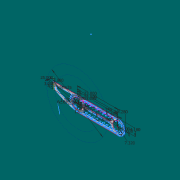
# Autodesk Inventor part: TG2
Saved by Autodesk Inventor 2016 (Build 200138000, 138)
## iProperties
Created: 2017-06-03
Part Number: TG2
Material: Aluminum 6061
Document SubType Name: Sheet Metal
Designer: katzchristy
Density: 2.7 g/cm^3
Appearance: Aluminum - Flat
Sheet Metal Rule: Default
Author: katzchristy
Autodesk Inventor part; units mm, degrees
ref_plane "YZ Plane" through (0, 0, 0) normal (1, 0, 0) x (0, 1, 0)
ref_plane "XZ Plane" through (0, 0, 0) normal (0, 1, 0) x (-1, 0, 0)
ref_plane "XY Plane" through (0, 0, 0) normal (0, 0, 1) x (1, 0, 0)
sketch "Fender Base" plane through (0, 0, 0) normal (0, 0, 1) x (1, 0, 0)
  line L0 (-7.62, 106.172) -> (7.62, 106.172) construction
  line L1 (111.252, 7.62) -> (111.252, -7.62)
  line L2 (576.58, 106.172) -> (591.82, 106.172) construction
  line L3 (692.912, 7.62) -> (692.912, -7.62) construction
  line L4 (-7.62, 106.172) -> (591.82, 106.172)
  arc A0 (528.4894, 74.422) -> (584.2, 92.964) centre (584.2, 0) ccw construction
  circle A1 centre (0, 0) radius 92.964 construction
  arc A2 (584.2, -106.4451) -> (591.82, 106.172) centre (584.2, 0) ccw
  line L5 (584.2, 0) -> (584.2, -74.422) construction
  line L6 (0, 0) -> (0, -106.4451) construction
  line L7 (0, -106.4451) -> (584.2, -106.4451)
  line L8 (0, 92.964) -> (584.2, 92.964) construction
  line L9 (0, -92.964) -> (584.2, -92.964) construction
  line L10 (75.7223, 74.422) -> (508.4777, 74.422)
  line L11 (0, 0) -> (584.2, 0) construction
  line L12 (75.7223, -74.422) -> (508.4777, -74.422)
  arc A3 (0, -74.422) -> (0, 74.422) centre (0, 0) ccw
  arc A4 (509.778, 0) -> (584.2, -74.422) centre (584.2, 0) ccw
  arc A5 (0, 74.422) -> (0, -74.422) centre (0, 0) ccw
  line L13 (584.2, -74.422) -> (584.2, -106.4451) construction
  arc A6 (584.2, 74.422) -> (509.778, 0) centre (584.2, 0) ccw
  arc A7 (584.2, -74.422) -> (584.2, 74.422) centre (584.2, 0) ccw
  arc A8 (479.2215, -15.875) -> (508.4777, -74.422) centre (584.2, 0) ccw
  arc A9 (508.4777, 74.422) -> (479.2215, 15.875) centre (584.2, 0) ccw
  arc A10 (584.2, 92.964) -> (528.4894, 74.422) centre (584.2, 0) ccw construction
  line L14 (104.9785, 15.875) -> (479.2215, 15.875)
  line L15 (104.9785, -15.875) -> (479.2215, -15.875)
  arc A11 (75.7223, -74.422) -> (104.9785, -15.875) centre (0, 0) ccw
  arc A12 (104.9785, 15.875) -> (75.7223, 74.422) centre (0, 0) ccw
  line L16 (111.252, 7.62) -> (111.252, -7.62) construction
  circle A13 centre (0, 0) radius 78.74 construction
  circle A14 centre (-433.085, 76.2) radius 38.1 construction
  circle A15 centre (0, 0) radius 439.7375 construction
  circle A16 centre (-306.5807, 82.55) radius 3.175 construction
  arc A17 (-317.4589, 5.1115) -> (-308.6545, 74.422) centre (0, 0) ccw construction
  line L17 (-429.979, 114.1732) -> (6.4191, 78.4779) construction
  line L18 (-443.1268, 39.4471) -> (-20.753, -75.9559) construction
  line L19 (-7.62, 106.172) -> (-347.8163, 106.172)
  line L20 (-347.8163, 155.9143) -> (-347.8163, -18.2544) construction
  arc A18 (-321.9776, 6.3462) -> (-34.5848, -100.67) centre (194.8237, 954.8143) ccw
  line L21 (-347.8163, 106.172) -> (-321.9776, 6.3462)
  line L22 (-283.1615, -143.6169) -> (-252.5039, -262.0603)
  arc A19 (-294.7226, 27.7545) -> (-91.9832, -53.5691) centre (194.8237, 954.8143) ccw
  line L23 (-294.7226, 27.7545) -> (-306.8019, 74.422)
  line L24 (-306.8019, 74.422) -> (-76.1047, 74.422)
  arc A20 (-76.1047, 74.422) -> (-91.9832, -53.5691) centre (0, 0) ccw
  arc A21 (-34.5848, -100.67) -> (0, -106.4451) centre (0, 0) ccw
  point P0 (0, 106.172)
  point P1 (111.252, 0)
  point P2 (584.2, 106.172)
  point P3 (692.912, 0)
  dimension "d100" = 879.475
  dimension "d0" = 15.24
  dimension "d1" = 106.172
  dimension "d2" = 15.24
  dimension "d3" = 111.252
  dimension "d4" = 15.24
  dimension "d5" = 106.172
  dimension "d6" = 584.2
  dimension "d7" = 15.24
  dimension "d8" = 108.712
  dimension "d9" = 584.2
  dimension "d10" = 185.928
  dimension "d11" = 185.928
  dimension "d13" = 584.2
  dimension "d14" = 31.75
  dimension "d66" = 31.75
  dimension "d96" = 157.48
  dimension "d97" = 76.2
  dimension "d99" = 76.2
  dimension "d101" = 6.35
  dimension "d102" = 82.55
  dimension "d103" = 635
  dimension "d106" = 31.75
  constraints: 50 end point, 43 point on circle, 21 centre point, 9 coincident, 8 point on line, 7 horizontal, 6 vertical, 5 tangent, 4 midpoint, 3 horizontal alignment, 2 equal length, 2 symmetric about line, 2 vertical alignment, 4 other
  measures "d0" distance of L0.start L0.end
  measures "d1" distance from line of point (0, 0) L0
  measures "d2" distance of L1.start L1.end
  measures "d3" distance from line of point (0, 0) L1
  measures "d4" distance of L2.start L2.end
  measures "d5" distance from line of point (0, 0) L2
  measures "d6" horizontal distance of point (0, 0) point (584.2, 106.172)
  measures "d7" distance of L3.start L3.end
  measures "d8" distance from line of L3 point (584.2, 0)
  measures "d9" distance of point (584.2, 0) point (0, 0)
  measures "d10" diameter of A0
  measures "d11" diameter of A1
  measures "d13" distance of A3.end A6.start
  measures "d14" distance between parallel lines of L10 L2
  measures "d66" distance between parallel lines of L15 L14
  measures "d96" diameter of A13
  measures "d97" diameter of A14
  measures "d99" vertical distance of point (0, 0) A14.centre
  measures "d101" diameter of A16
  measures "d102" vertical distance of point (0, 0) A16.centre
  measures "d103" diameter of A17
  measures "d106" radial gap between concentric circles of A18 A19
extrude "Plate1" add sketch "Fender Base" along normal blind 1.6281 contours L4 A2 L7 A21 A18 L21 L19 | L10 A9 L14 A12 | A5 A3 | A6 A7 A4 | L23 L24 A20 A19
sketch "Oval Pattern" plane through (0, 0, 1.6281) normal (0, 0, 1) x (1, 0, 0)
  circle A0 centre (-25.6073, 82.042) radius 6.35
  arc A1 (-14.4463, 83.0479) -> (-28.9236, 92.7462) centre (-25.6073, 82.042) ccw
  arc A2 (12.2648, 98.9975) -> (-28.9236, 92.7462) centre (-1.2605, 49.2962) ccw
  arc A3 (12.2648, 98.9975) -> (-14.4463, 83.0479) centre (17.7837, 59.4132) ccw
  circle A4 centre (-61.4767, 60.0603) radius 6.35
  arc A5 (-52.1303, 66.2426) -> (-69.4759, 67.9082) centre (-61.4767, 60.0603) ccw
  arc A6 (-36.1888, 92.9586) -> (-69.4759, 67.9082) centre (-24.5055, 42.7924) ccw
  arc A7 (-36.1888, 92.9586) -> (-52.1303, 66.2426) centre (-12.5443, 60.7357) ccw
  circle A8 centre (-82.6165, 23.6883) radius 6.35
  arc A9 (-77.3239, 33.5658) -> (-93.3821, 26.7996) centre (-82.6165, 23.6883) ccw
  arc A10 (-75.9716, 64.6471) -> (-93.3821, 26.7996) centre (-41.879, 26.0356) ccw
  arc A11 (-75.9716, 64.6471) -> (-77.3239, 33.5658) centre (-39.8667, 47.5062) ccw
  circle A12 centre (-83.9616, -18.3594) radius 6.35
  arc A13 (-83.991, -7.1533) -> (-94.9141, -20.7301) centre (-83.9616, -18.3594) ccw
  arc A14 (-97.5518, 20.8463) -> (-94.9141, -20.7301) centre (-49.2185, 3.0408) ccw
  arc A15 (-97.5518, 20.8463) -> (-83.991, -7.1533) centre (-57.6371, 22.8943) ccw
  circle A16 centre (-65.1898, -56.0082) radius 6.35
  arc A17 (-70.534, -46.1585) -> (-73.705, -63.293) centre (-65.1898, -56.0082) ccw
  arc A18 (-95.7589, -27.9492) -> (-73.705, -63.293) centre (-44.7653, -20.6826) ccw
  arc A19 (-95.7589, -27.9492) -> (-70.534, -46.1585) centre (-61.5979, -7.2031) ccw
  circle A20 centre (-30.7986, -80.2376) radius 6.35
  arc A21 (-40.1773, -74.1042) -> (-34.8364, -90.691) centre (-30.7986, -80.2376) ccw
  arc A22 (-71.0224, -70.0481) -> (-34.8364, -90.691) centre (-29.5865, -39.4505) ccw
  arc A23 (-71.0224, -70.0481) -> (-40.1773, -74.1042) centre (-50.8, -35.5745) ccw
  circle A24 centre (10.9718, -85.2423) radius 6.35
  arc A25 (-0.1943, -84.2948) -> (12.3789, -96.3597) centre (10.9718, -85.2423) ccw
  arc A26 (-29.2692, -95.3637) -> (12.3789, -96.3597) centre (-7.3189, -48.7662) ccw
  arc A27 (-29.2692, -95.3637) -> (-0.1943, -84.2948) centre (-27.8305, -55.4225) ccw
  line L0 (-347.8163, 106.172) -> (591.82, 106.172) projected
  circle A28 centre (19.9908, 83.9489) radius 6.35
  arc A29 (31.1517, 84.9548) -> (16.6745, 94.6531) centre (19.9908, 83.9489) ccw
  arc A30 (57.8628, 100.9043) -> (16.6745, 94.6531) centre (44.3376, 51.2031) ccw
  arc A31 (57.8628, 100.9043) -> (31.1517, 84.9548) centre (63.3817, 61.32) ccw
  circle A32 centre (65.7108, 83.9489) radius 6.35
  arc A33 (76.8717, 84.9548) -> (62.3945, 94.6531) centre (65.7108, 83.9489) ccw
  arc A34 (103.5828, 100.9043) -> (76.8717, 84.9548) centre (109.1017, 61.32) ccw
  arc A35 (103.5828, 100.9043) -> (62.3945, 94.6531) centre (90.0576, 51.2031) ccw
  circle A36 centre (111.4308, 83.9489) radius 6.35
  arc A37 (122.5917, 84.9548) -> (108.1145, 94.6531) centre (111.4308, 83.9489) ccw
  arc A38 (149.3028, 100.9043) -> (122.5917, 84.9548) centre (154.8217, 61.32) ccw
  arc A39 (149.3028, 100.9043) -> (108.1145, 94.6531) centre (135.7776, 51.2031) ccw
  circle A40 centre (157.1508, 83.9489) radius 6.35
  arc A41 (168.3117, 84.9548) -> (153.8345, 94.6531) centre (157.1508, 83.9489) ccw
  arc A42 (195.0228, 100.9043) -> (168.3117, 84.9548) centre (200.5417, 61.32) ccw
  arc A43 (195.0228, 100.9043) -> (153.8345, 94.6531) centre (181.4976, 51.2031) ccw
  circle A44 centre (202.8708, 83.9489) radius 6.35
  arc A45 (214.0317, 84.9548) -> (199.5545, 94.6531) centre (202.8708, 83.9489) ccw
  arc A46 (240.7428, 100.9043) -> (214.0317, 84.9548) centre (246.2617, 61.32) ccw
  arc A47 (240.7428, 100.9043) -> (199.5545, 94.6531) centre (227.2176, 51.2031) ccw
  circle A48 centre (248.5908, 83.9489) radius 6.35
  arc A49 (259.7517, 84.9548) -> (245.2745, 94.6531) centre (248.5908, 83.9489) ccw
  arc A50 (286.4628, 100.9043) -> (259.7517, 84.9548) centre (291.9817, 61.32) ccw
  arc A51 (286.4628, 100.9043) -> (245.2745, 94.6531) centre (272.9376, 51.2031) ccw
  circle A52 centre (294.3108, 83.9489) radius 6.35
  arc A53 (305.4717, 84.9548) -> (290.9945, 94.6531) centre (294.3108, 83.9489) ccw
  arc A54 (332.1828, 100.9043) -> (305.4717, 84.9548) centre (337.7017, 61.32) ccw
  arc A55 (332.1828, 100.9043) -> (290.9945, 94.6531) centre (318.6576, 51.2031) ccw
  circle A56 centre (340.0308, 83.9489) radius 6.35
  arc A57 (351.1917, 84.9548) -> (336.7145, 94.6531) centre (340.0308, 83.9489) ccw
  arc A58 (377.9028, 100.9043) -> (351.1917, 84.9548) centre (383.4217, 61.32) ccw
  arc A59 (377.9028, 100.9043) -> (336.7145, 94.6531) centre (364.3776, 51.2031) ccw
  circle A60 centre (385.7508, 83.9489) radius 6.35
  arc A61 (396.9117, 84.9548) -> (382.4345, 94.6531) centre (385.7508, 83.9489) ccw
  arc A62 (423.6228, 100.9043) -> (396.9117, 84.9548) centre (429.1417, 61.32) ccw
  arc A63 (423.6228, 100.9043) -> (382.4345, 94.6531) centre (410.0976, 51.2031) ccw
  circle A64 centre (431.4708, 83.9489) radius 6.35
  arc A65 (442.6317, 84.9548) -> (428.1545, 94.6531) centre (431.4708, 83.9489) ccw
  arc A66 (469.3428, 100.9043) -> (442.6317, 84.9548) centre (474.8617, 61.32) ccw
  arc A67 (469.3428, 100.9043) -> (428.1545, 94.6531) centre (455.8176, 51.2031) ccw
  circle A68 centre (477.1908, 83.9489) radius 6.35
  arc A69 (488.3517, 84.9548) -> (473.8745, 94.6531) centre (477.1908, 83.9489) ccw
  arc A70 (515.0628, 100.9043) -> (488.3517, 84.9548) centre (520.5817, 61.32) ccw
  arc A71 (515.0628, 100.9043) -> (473.8745, 94.6531) centre (501.5376, 51.2031) ccw
  circle A72 centre (522.9108, 83.9489) radius 6.35
  arc A73 (534.0717, 84.9548) -> (519.5945, 94.6531) centre (522.9108, 83.9489) ccw
  arc A74 (560.7828, 100.9043) -> (534.0717, 84.9548) centre (566.3017, 61.32) ccw
  arc A75 (560.7828, 100.9043) -> (519.5945, 94.6531) centre (547.2576, 51.2031) ccw
  circle A76 centre (568.6308, 83.9489) radius 6.35
  arc A77 (579.7917, 84.9548) -> (565.3145, 94.6531) centre (568.6308, 83.9489) ccw
  arc A78 (606.5028, 100.9043) -> (579.7917, 84.9548) centre (612.0217, 61.32) ccw
  arc A79 (606.5028, 100.9043) -> (565.3145, 94.6531) centre (592.9776, 51.2031) ccw
  line L1 (75.7223, 74.422) -> (508.4777, 74.422) projected
  circle A80 centre (612.6911, 80.4865) radius 6.35
  arc A81 (622.8597, 75.7771) -> (615.1712, 91.4147) centre (612.6911, 80.4865) ccw
  arc A82 (653.967, 76.2343) -> (615.1712, 91.4147) centre (617.4031, 39.9544) ccw
  arc A83 (653.967, 76.2343) -> (622.8597, 75.7771) centre (638.9544, 39.1938) ccw
  circle A84 centre (649.1172, 55.4578) radius 6.35
  arc A85 (655.5688, 46.2951) -> (656.7292, 63.6819) centre (649.1172, 55.4578) ccw
  arc A86 (682.7371, 31.1374) -> (656.7292, 63.6819) centre (632.9319, 17.9999) ccw
  arc A87 (682.7371, 31.1374) -> (655.5688, 46.2951) centre (651.2156, 6.5657) ccw
  circle A88 centre (668.1489, 15.5692) radius 6.35
  arc A89 (669.1548, 4.4083) -> (678.8531, 18.8855) centre (668.1489, 15.5692) ccw
  arc A90 (685.1043, -22.3028) -> (678.8531, 18.8855) centre (635.4031, -8.7776) ccw
  arc A91 (685.1043, -22.3028) -> (669.1548, 4.4083) centre (645.52, -27.8217) ccw
  circle A92 centre (664.6865, -28.4911) radius 6.35
  arc A93 (659.9771, -38.6597) -> (675.6147, -30.9712) centre (664.6865, -28.4911) ccw
  arc A94 (660.4343, -69.767) -> (675.6147, -30.9712) centre (624.1544, -33.2031) ccw
  arc A95 (660.4343, -69.767) -> (659.9771, -38.6597) centre (623.3938, -54.7544) ccw
  circle A96 centre (639.6578, -64.9172) radius 6.35
  arc A97 (630.4951, -71.3688) -> (647.8819, -72.5292) centre (639.6578, -64.9172) ccw
  arc A98 (615.3374, -98.5371) -> (647.8819, -72.5292) centre (602.1999, -48.7319) ccw
  arc A99 (615.3374, -98.5371) -> (630.4951, -71.3688) centre (590.7657, -67.0156) ccw
  circle A100 centre (599.7692, -83.9489) radius 6.35
  arc A101 (588.6083, -84.9548) -> (603.0855, -94.6531) centre (599.7692, -83.9489) ccw
  arc A102 (561.8972, -100.9043) -> (603.0855, -94.6531) centre (575.4224, -51.2031) ccw
  arc A103 (561.8972, -100.9043) -> (588.6083, -84.9548) centre (556.3783, -61.32) ccw
  line L2 (584.2, -106.4451) -> (0, -106.4451) projected
  circle A104 centre (60.5018, -85.2423) radius 6.35
  arc A105 (49.3357, -84.2948) -> (61.9089, -96.3597) centre (60.5018, -85.2423) ccw
  arc A106 (20.2608, -95.3637) -> (49.3357, -84.2948) centre (21.6995, -55.4225) ccw
  arc A107 (20.2608, -95.3637) -> (61.9089, -96.3597) centre (42.2111, -48.7662) ccw
  circle A108 centre (110.0318, -85.2423) radius 6.35
  arc A109 (98.8657, -84.2948) -> (111.4389, -96.3597) centre (110.0318, -85.2423) ccw
  arc A110 (69.7908, -95.3637) -> (98.8657, -84.2948) centre (71.2295, -55.4225) ccw
  arc A111 (69.7908, -95.3637) -> (111.4389, -96.3597) centre (91.7411, -48.7662) ccw
  circle A112 centre (159.5618, -85.2423) radius 6.35
  arc A113 (148.3957, -84.2948) -> (160.9689, -96.3597) centre (159.5618, -85.2423) ccw
  arc A114 (119.3208, -95.3637) -> (148.3957, -84.2948) centre (120.7595, -55.4225) ccw
  arc A115 (119.3208, -95.3637) -> (160.9689, -96.3597) centre (141.2711, -48.7662) ccw
  circle A116 centre (209.0918, -85.2423) radius 6.35
  arc A117 (197.9257, -84.2948) -> (210.4989, -96.3597) centre (209.0918, -85.2423) ccw
  arc A118 (168.8508, -95.3637) -> (197.9257, -84.2948) centre (170.2895, -55.4225) ccw
  arc A119 (168.8508, -95.3637) -> (210.4989, -96.3597) centre (190.8011, -48.7662) ccw
  circle A120 centre (258.6218, -85.2423) radius 6.35
  arc A121 (247.4557, -84.2948) -> (260.0289, -96.3597) centre (258.6218, -85.2423) ccw
  arc A122 (218.3808, -95.3637) -> (247.4557, -84.2948) centre (219.8195, -55.4225) ccw
  arc A123 (218.3808, -95.3637) -> (260.0289, -96.3597) centre (240.3311, -48.7662) ccw
  circle A124 centre (308.1518, -85.2423) radius 6.35
  arc A125 (296.9857, -84.2948) -> (309.5589, -96.3597) centre (308.1518, -85.2423) ccw
  arc A126 (267.9108, -95.3637) -> (296.9857, -84.2948) centre (269.3495, -55.4225) ccw
  arc A127 (267.9108, -95.3637) -> (309.5589, -96.3597) centre (289.8611, -48.7662) ccw
  circle A128 centre (357.6818, -85.2423) radius 6.35
  arc A129 (346.5157, -84.2948) -> (359.0889, -96.3597) centre (357.6818, -85.2423) ccw
  arc A130 (317.4408, -95.3637) -> (346.5157, -84.2948) centre (318.8795, -55.4225) ccw
  arc A131 (317.4408, -95.3637) -> (359.0889, -96.3597) centre (339.3911, -48.7662) ccw
  circle A132 centre (407.2118, -85.2423) radius 6.35
  arc A133 (396.0457, -84.2948) -> (408.6189, -96.3597) centre (407.2118, -85.2423) ccw
  arc A134 (366.9708, -95.3637) -> (396.0457, -84.2948) centre (368.4095, -55.4225) ccw
  arc A135 (366.9708, -95.3637) -> (408.6189, -96.3597) centre (388.9211, -48.7662) ccw
  circle A136 centre (456.7418, -85.2423) radius 6.35
  arc A137 (445.5757, -84.2948) -> (458.1489, -96.3597) centre (456.7418, -85.2423) ccw
  arc A138 (416.5008, -95.3637) -> (445.5757, -84.2948) centre (417.9395, -55.4225) ccw
  arc A139 (416.5008, -95.3637) -> (458.1489, -96.3597) centre (438.4511, -48.7662) ccw
  circle A140 centre (506.2718, -85.2423) radius 6.35
  arc A141 (495.1057, -84.2948) -> (507.6789, -96.3597) centre (506.2718, -85.2423) ccw
  arc A142 (466.0308, -95.3637) -> (495.1057, -84.2948) centre (467.4695, -55.4225) ccw
  arc A143 (466.0308, -95.3637) -> (507.6789, -96.3597) centre (487.9811, -48.7662) ccw
  circle A144 centre (555.8018, -85.2423) radius 6.35
  arc A145 (544.6357, -84.2948) -> (557.2089, -96.3597) centre (555.8018, -85.2423) ccw
  arc A146 (515.5608, -95.3637) -> (544.6357, -84.2948) centre (516.9995, -55.4225) ccw
  arc A147 (515.5608, -95.3637) -> (557.2089, -96.3597) centre (537.5111, -48.7662) ccw
  line L3 (104.9785, 15.875) -> (479.2215, 15.875) projected
  arc A148 (104.9785, 15.875) -> (75.7223, 74.422) centre (0, 0) ccw projected
  arc A149 (508.4777, 74.422) -> (479.2215, 15.875) centre (584.2, 0) ccw projected
  circle A150 centre (430.2676, 0) radius 8.89
  line L4 (0, 0) -> (584.2, 0) construction
  line L5 (430.2676, 8.89) -> (430.2676, -8.89) construction
  arc A151 (423.8766, 11.8482) -> (423.8766, -11.8482) centre (430.2676, 0) ccw
  arc A152 (436.6586, -11.8482) -> (436.6586, 11.8482) centre (430.2676, 0) ccw
  arc A153 (423.8766, 11.8482) -> (389.1564, 0) centre (441.3857, -96.257) ccw
  arc A154 (389.1564, 0) -> (423.8766, -11.8482) centre (441.3857, 96.257) ccw
  arc A155 (471.3788, 0) -> (436.6586, 11.8482) centre (419.1495, -96.257) ccw
  arc A156 (436.6586, -11.8482) -> (471.3788, 0) centre (419.1495, 96.257) ccw
  arc A157 (584.2, 74.422) -> (509.778, 0) centre (584.2, 0) ccw projected
  arc A158 (509.778, 0) -> (584.2, -74.422) centre (584.2, 0) ccw projected
  arc A159 (0, 74.422) -> (0, -74.422) centre (0, 0) ccw projected
  arc A160 (0, -74.422) -> (0, 74.422) centre (0, 0) ccw projected
  arc A161 (75.7223, -74.422) -> (104.9785, -15.875) centre (0, 0) ccw construction
  arc A162 (300.2564, 0) -> (334.9766, -11.8482) centre (352.4857, 96.257) ccw
  arc A163 (334.9766, 11.8482) -> (300.2564, 0) centre (352.4857, -96.257) ccw
  arc A164 (334.9766, 11.8482) -> (334.9766, -11.8482) centre (341.3676, 0) ccw
  line L6 (341.3676, 8.89) -> (341.3676, -8.89) construction
  circle A165 centre (341.3676, 0) radius 8.89
  arc A166 (347.7586, -11.8482) -> (347.7586, 11.8482) centre (341.3676, 0) ccw
  arc A167 (382.4788, 0) -> (347.7586, 11.8482) centre (330.2495, -96.257) ccw
  arc A168 (347.7586, -11.8482) -> (382.4788, 0) centre (330.2495, 96.257) ccw
  arc A169 (211.3564, 0) -> (246.0766, -11.8482) centre (263.5857, 96.257) ccw
  arc A170 (246.0766, 11.8482) -> (211.3564, 0) centre (263.5857, -96.257) ccw
  arc A171 (246.0766, 11.8482) -> (246.0766, -11.8482) centre (252.4676, 0) ccw
  line L7 (252.4676, 8.89) -> (252.4676, -8.89) construction
  circle A172 centre (252.4676, 0) radius 8.89
  arc A173 (258.8586, -11.8482) -> (258.8586, 11.8482) centre (252.4676, 0) ccw
  arc A174 (293.5788, 0) -> (258.8586, 11.8482) centre (241.3495, -96.257) ccw
  arc A175 (258.8586, -11.8482) -> (293.5788, 0) centre (241.3495, 96.257) ccw
  arc A176 (122.4564, 0) -> (157.1766, -11.8482) centre (174.6857, 96.257) ccw
  arc A177 (157.1766, 11.8482) -> (122.4564, 0) centre (174.6857, -96.257) ccw
  arc A178 (157.1766, 11.8482) -> (157.1766, -11.8482) centre (163.5676, 0) ccw
  line L8 (163.5676, 8.89) -> (163.5676, -8.89) construction
  circle A179 centre (163.5676, 0) radius 8.89
  arc A180 (169.9586, -11.8482) -> (169.9586, 11.8482) centre (163.5676, 0) ccw
  arc A181 (204.6788, 0) -> (169.9586, 11.8482) centre (152.4495, -96.257) ccw
  arc A182 (169.9586, -11.8482) -> (204.6788, 0) centre (152.4495, 96.257) ccw
  line L9 (88.6116, 11.43) -> (116.3818, 11.43)
  line L10 (116.3818, 11.43) -> (116.3818, -11.43)
  line L11 (116.3818, -11.43) -> (88.6116, -11.43)
  line L12 (88.6116, -11.43) -> (88.6116, 11.43)
  line L13 (110.6883, 7.3883) -> (110.6883, -7.6711) construction
  point P0 (-7.62, 106.172)
  point P1 (9.4092, 94.8654)
  point P2 (614.3723, 99.0943)
  point P3 (659.8771, 70.7321)
  point P4 (685.1043, 23.4172)
  point P5 (683.2943, -30.1723)
  point P6 (654.9321, -75.6771)
  point P7 (607.6172, -100.9043)
  point P8 (116.3818, 0)
  dimension "d38" = 170
  dimension "d44" = 45.72
  dimension "d51" = 180
  dimension "d55" = 49.53
  dimension "d69" = 17.78
  dimension "d87" = 88.9
  dimension "d92" = 22.86
  dimension "d94" = 5.6935
  constraints: 278 point on circle, 176 centre point, 18 end point, 7 symmetric about line, 4 horizontal, 2 parallel, 1 horizontal alignment, 1 midpoint, 1 perpendicular, 1 vertical, 458 other
  measures "d44" distance of A28.centre A32.centre
  measures "d55" distance of A24.centre A104.centre
  measures "d69" diameter of A150
  measures "d87" distance of A151.end A162.end
  measures "d92" distance of L11.end L9.start
  measures "d94" distance between parallel lines of L13 L10
extrude "Cut1" cut sketch "Fender Base" along normal through all contours A5 A3
extrude "Cut2" cut sketch "Fender Base" along normal through all contours A6 A7 A4
extrude "Cut3" cut sketch "Fender Base" along normal through all contours L10 A9 L14 A12
extrude "Cut4" cut sketch "Fender Base" along normal through all contours L23 L24 A20 A19
equation "\"d11\" = d10"
equation "\"d62\" = Thickness"
equation "\"d64\" = Thickness"
equation "\"d67\" = Thickness"
equation "\"BendRadius\" = Thickness"
equation "\"BendReliefWidth\" = Thickness"
equation "\"BendReliefDepth\" = 0.5 * Thickness"
equation "\"CornerReliefSize\" = 4 * Thickness"
equation "\"MinimumRemnant\" = 2 * Thickness"
equation "\"TransitionRadius\" = BendRadius"
equation "\"JacobiRadiusSize\" = Thickness"
equation "\"GapSize\" = Thickness"
equation "\"d23\" = BendRadius"
equation "\"Thickness\" = 1.62814"
body "Solid1"
